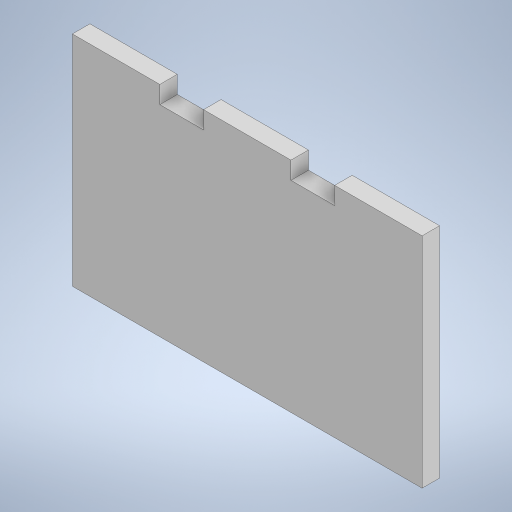
# Autodesk Inventor part: стенка
Saved by Autodesk Inventor 2023 (Build 270158000, 158)
## iProperties
Created: 2025-02-04
Part Number: стенка
Material: Типовые
Document SubType Name: Modeling
Designer: baranovaem
Density: 1 g/cm^3
Appearance: По умолчанию
Author: baranovaem
Autodesk Inventor part; units mm, degrees
ref_plane "YZ Plane" through (0, 0, 0) normal (1, 0, 0) x (0, 1, 0)
ref_plane "XZ Plane" through (0, 0, 0) normal (0, 1, 0) x (-1, 0, 0)
ref_plane "XY Plane" through (0, 0, 0) normal (0, 0, 1) x (1, 0, 0)
sketch "Эскиз1" plane through (0, 0, 0) normal (0, 0, 1) x (1, 0, 0)
  line L0 (-40, 23) -> (40, 23)
  line L1 (40, 23) -> (40, -23)
  line L2 (40, -23) -> (-40, -23)
  line L3 (-40, -23) -> (-40, 23)
  line L4 (-40, 23) -> (40, -23) construction
  line L5 (40, 23) -> (-40, -23) construction
  point P0 (0, 0)
  dimension "d0" = 80
  dimension "d1" = 46
  constraints: 12 end point, 2 midpoint, 2 parallel, 1 horizontal, 1 perpendicular
  measures "d0" distance of L1.end L2.end
  measures "d1" distance of L0.end L1.end
extrude "Выдавливание1" add sketch "Эскиз1" along normal blind 4
sketch "Эскиз2" plane through (-40, 23, 0) normal (0, 1, 0) x (1, 0, 0)
  line L0 (0, -4) -> (80, -4) projected
  line L1 (0, 0) -> (80, 0) projected
  line L2 (0, -4) -> (20, -4)
  line L3 (20, -4) -> (20, 0)
  line L4 (20, 0) -> (0, 0)
  line L5 (0, 0) -> (0, -4)
  line L6 (80, -4) -> (60, -4)
  line L7 (60, -4) -> (60, 0)
  line L8 (60, 0) -> (80, 0)
  line L9 (80, 0) -> (80, -4)
  line L10 (50, -4) -> (30, -4)
  line L11 (30, -4) -> (30, 0)
  line L12 (30, 0) -> (50, 0)
  line L13 (50, 0) -> (50, -4)
  point P0 (40, 0)
  point P1 (30, -2)
  point P2 (20, -2)
  point P3 (60, -2)
  point P4 (50, -2)
  dimension "d4" = 10
  dimension "d6" = 20
  constraints: 24 end point, 6 parallel, 5 point on line, 4 midpoint, 3 horizontal, 3 perpendicular
  measures "d4" distance of point (30, -2) point (20, -2)
  measures "d6" distance of point (50, -2) point (30, -2)
extrude "Выдавливание2" add sketch "Эскиз2" along normal blind 4 contours L5 L1 L3 L0 | L11 L1 L13 L0 | L7 L1 L9 L0
